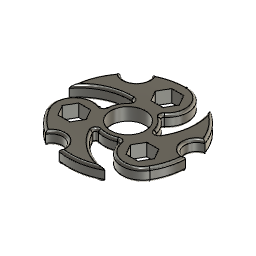
fidget_spinner (Autodesk Fusion 360 design; units mm, degrees)
Autodesk Fusion 360 part; units mm, degrees
sketch "Sketch1" plane through (0, 0, 0) normal (0, 0, 1) x (1, 0, 0)
  circle A0 centre (0, 0) radius 45 construction
  circle A1 centre (0, 0) radius 11
  circle A2 centre (0, 0) radius 15
  circle A3 centre (0, 25) radius 13
  line L0 (-3.8105, 31.6) -> (-7.621, 25)
  line L1 (-7.621, 25) -> (-3.8105, 18.4)
  line L2 (-3.8105, 18.4) -> (3.8105, 18.4)
  line L3 (3.8105, 18.4) -> (7.621, 25)
  line L4 (7.621, 25) -> (3.8105, 31.6)
  line L5 (3.8105, 31.6) -> (-3.8105, 31.6)
  circle A4 centre (0, 25) radius 9
  line L6 (0, 25) -> (9, 25) construction
  circle A5 centre (0, 0) radius 38
  line L7 (0, 25) -> (0, 38) construction
  arc A6 (-3.4205, 12.4581) -> (-37.9938, 0.686) centre (-12, -19) ccw
  circle A7 centre (-24, 29.4618) radius 7.5
  circle A8 centre (-21.6506, -12.5) radius 13
  circle A9 centre (-21.6506, -12.5) radius 9
  line L8 (-25.4611, -19.1) -> (-17.8401, -19.1)
  line L9 (-29.2717, -12.5) -> (-25.4611, -19.1)
  line L10 (-25.4611, -5.9) -> (-29.2717, -12.5)
  line L11 (-17.8401, -5.9) -> (-25.4611, -5.9)
  line L12 (-14.0296, -12.5) -> (-17.8401, -5.9)
  line L13 (-17.8401, -19.1) -> (-14.0296, -12.5)
  arc A10 (-9.0787, -9.1913) -> (18.4028, -33.2466) centre (22.4545, -0.8923) ccw
  circle A11 centre (-13.5147, -35.5155) radius 7.5
  circle A12 centre (21.6506, -12.5) radius 13
  circle A13 centre (21.6506, -12.5) radius 9
  line L14 (29.2717, -12.5) -> (25.4611, -5.9)
  line L15 (25.4611, -19.1) -> (29.2717, -12.5)
  line L16 (17.8401, -19.1) -> (25.4611, -19.1)
  line L17 (14.0296, -12.5) -> (17.8401, -19.1)
  line L18 (17.8401, -5.9) -> (14.0296, -12.5)
  line L19 (25.4611, -5.9) -> (17.8401, -5.9)
  arc A14 (12.4993, -3.2668) -> (19.591, 32.5606) centre (-10.4545, 19.8923) ccw
  circle A15 centre (37.5147, 6.0537) radius 7.5
  point P0 (0, 25)
  dimension "d1" = 90
  dimension "d2" = 22
  dimension "d3" = 30
  dimension "d5" = 6.6
  dimension "d6" = 18
  dimension "d7" = 26
  dimension "d8" = 25
  dimension "d9" = 19
  dimension "d10" = 12
  dimension "d11" = 32.607
  dimension "d12" = 15
  dimension "d13" = 24
  dimension "d15" = 360
  constraint coincident A0.centre A1.centre
  constraint coincident P0 A3.centre
  constraint concentric A3 A4
  constraint vertical A0.centre P0
  constraint coincident A4 L6.end
  constraint horizontal L6
  constraint coincident L3.end L6
  constraint coincident A3 L7.end
  constraint vertical L7
  constraint coincident A5 L7.end
  constraint coincident A5 A6.end
  constraint coincident A3 A6.start
  constraint coincident A5 A7.centre
  measures "d1" diameter of A0
  measures "d2" diameter of A1
  measures "d3" diameter of A2
  measures "d5" distance of P0 L5
  measures "d6" diameter of A4
  measures "d7" diameter of A3
  measures "d8" distance of A0.centre P0
  measures "d9" vertical distance of A0.centre A6.centre
  measures "d10" horizontal distance of A0.centre A6.centre
  measures "d11" radius of A6
  measures "d12" diameter of A7
  measures "d13" horizontal distance of A0.centre A7.centre
extrude "Extrude1" add sketch "Sketch1" along normal blind 8 contours A2 A3 A6 A8 A10 A12 A14 | A2 A3 | A2 A3 | A2 A5 A12 A14 A15 | A2 A12 A14 | A2 A3 A6 | A2 A3 A5 A6 A7 | A2 A12 | A2 A12 | A2 A8 | A2 A8 | A2 A5 A8 A10 A11 | A2 A8 A10 | A4 | A9 | A13
mesh "Mesh1" [no effect]
fillet "Fillet1" radius 1.5 6 edges at (-7.9259, -12.735, 4) (8.653, -12.2526, 4) (-7.0659, 13.2315, 4) (-14.9375, -1.3674, 4) (14.9918, -0.4965, 4) (6.2846, 13.62, 4)
fillet "Fillet2" radius 1.5 48 edges at (22.0613, 17.4551, 8) (15.8447, 2.1886, 8) (12.345, 8.5206, 8) (7.6375, 13.6689, 8) (12.2523, 29.3453, 8) (-9.1415, 36.884, 8) (4.0859, -27.8332, 8) (-6.027, -14.8162, 8) (1.2066, -14.9514, 8) (8.0189, -13.4487, 8) (19.2876, -25.2834, 8) (36.5133, -10.5252, 8) (29.2247, 24.2883, 8) (30.1105, 4.8589, 8) (-26.1472, 10.3781, 8) (-9.8177, 12.6276, 8) (-13.5516, 6.4308, 8) (-15.6563, -0.2202, 8) (-31.5399, -4.0618, 8) (-27.3718, -26.3588, 8) (-10.8473, -28.5059, 8) (6.4219, -37.4534, 8) (-35.6466, 13.1652, 8) (-19.2632, 23.647, 8) (4.0859, -27.8332, 0) (-6.027, -14.8162, 0) (1.2066, -14.9514, 0) (8.0189, -13.4487, 0) (19.2876, -25.2834, 0) (36.5133, -10.5252, 0) (30.1105, 4.8589, 0) (29.2247, 24.2883, 0) (-9.1415, 36.884, 0) (12.2523, 29.3453, 0) (7.6375, 13.6689, 0) (12.345, 8.5206, 0) (15.8447, 2.1886, 0) (22.0613, 17.4551, 0) (-19.2632, 23.647, 0) (-35.6466, 13.1652, 0) (-27.3718, -26.3588, 0) (-31.5399, -4.0618, 0) (-15.6563, -0.2202, 0) (-13.5516, 6.4308, 0) (-9.8177, 12.6276, 0) (-26.1472, 10.3781, 0) (-10.8473, -28.5059, 0) (6.4219, -37.4534, 0)
